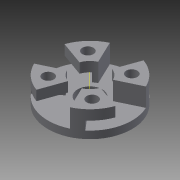
# Autodesk Inventor part: new male 4 bay con
Saved by Autodesk Inventor 2015 (Build 190159000, 159)
## iProperties
Created: 2014-11-16
Part Number: new male 4 bay con
Material: Generic
Document SubType Name: Modeling
Designer: ericd_000
Density: 1 g/cm^3
Appearance: Default
Author: ericd_000
Autodesk Inventor part; units mm, degrees
ref_plane "YZ Plane" through (0, 0, 0) normal (1, 0, 0) x (0, 1, 0)
ref_plane "XZ Plane" through (0, 0, 0) normal (0, 1, 0) x (-1, 0, 0)
ref_plane "XY Plane" through (0, 0, 0) normal (0, 0, 1) x (1, 0, 0)
sketch "Sketch1" plane through (0, 0, 0) normal (0, 0, 1) x (1, 0, 0)
  circle A0 centre (0, 0) radius 34
  dimension "d0" = 68
  constraints: 1 centre point, 1 coincident
  measures "d0" diameter of A0
extrude "Extrusion1" add sketch "Sketch1" along normal blind 6
sketch "Sketch2" plane through (0, 0, 6) normal (0, 0, 1) x (1, 0, 0)
  circle A0 centre (0, 0) radius 34
  circle A1 centre (0, 0) radius 34 projected
  line L0 (0, 0) -> (30.6997, 14.6126) construction
  line L1 (0, 0) -> (25.8716, 22.0604) construction
  line L2 (25.8716, 22.0604) -> (10.653, 9.0837)
  line L3 (30.6997, 14.6126) -> (12.641, 6.017)
  arc A2 (30.6997, 14.6126) -> (25.8716, 22.0604) centre (0, 0) ccw
  arc A3 (12.641, 6.017) -> (10.653, 9.0837) centre (0, 0) ccw
  dimension "d3" = 15
  dimension "d4" = 20
  constraints: 8 end point, 8 point on circle, 3 centre point, 3 concentric, 2 point on line, 1 coincident
  measures "d3" angle of L0 L1
  measures "d4" distance of L1.end L2.end
extrude "Extrusion2" add sketch "Sketch2" along normal blind 15 contours L3 A3 L2 A0 picked at (22.8031, 15.025)
sketch "Sketch3" plane through (10.653, 9.0837, 21) normal (-0.6488347, 0.7609293, 0) x (0.7609293, 0.6488347, 0)
  line L0 (0, 15) -> (0, 0) projected
  line L1 (20, 0) -> (0, 0)
  line L2 (0, 0) -> (0, 8)
  line L3 (0, 8) -> (20, 8)
  line L4 (20, 8) -> (20, 0)
  line L5 (-14, 25.2) -> (-14, -4.2) projected
  line L6 (-48, 15) -> (20, 15) projected
  point P0 (-14, 21)
  point P1 (18.8415, 15)
  dimension "d7" = 8
  dimension "d26" = 7
  constraints: 8 end point, 2 parallel, 1 horizontal, 1 perpendicular, 1 point on line
  measures "d7" distance between parallel lines of L3 L1
  measures "d26" distance between parallel lines of L6 L3
revolve "Revolution1" add sketch "Sketch3" angle 30 about axis through (0, 0, 6) along (0, 0, 1)
sketch "Sketch4" plane through (0, 0, 21) normal (0, 0, 1) x (1, 0, 0)
  circle A0 centre (16.0735, 17.8225) radius 4.5
  arc A1 (12.641, 6.017) -> (4.6839, 13.1932) centre (0, 0) ccw projected
  arc A2 (30.6997, 14.6126) -> (11.3753, 32.0406) centre (0, 0) ccw projected
  line L0 (12.641, 6.017) -> (30.6997, 14.6126) projected
  line L1 (4.6839, 13.1932) -> (11.3753, 32.0406) projected
  arc A3 (21.6704, 10.3148) -> (8.0296, 22.6169) centre (0, 0) ccw construction
  circle A4 centre (0, 0) radius 34 construction
  line L2 (22.7708, 25.2486) -> (18.7388, 20.7779) construction
  dimension "d12" = 9
  constraints: 5 point on circle, 2 centre point, 2 end point, 2 midpoint, 1 concentric, 1 line through centre, 1 point on line
  measures "d12" diameter of A0
extrude "Extrusion3" cut sketch "Sketch4" against normal blind 10 contours A0
pattern_circular "Circular Pattern2" count 4 over 360 about axis through (0, 0, 6) along (0, 0, 1) of "Revolution1", "Extrusion3", "Extrusion2"
sketch "Sketch5" plane through (0, 0, 0) normal (0, 0, -1) x (-1, 0, 0)
  circle A0 centre (0, 0) radius 10
  dimension "d23" = 20
  constraints: 1 centre point, 1 coincident
  measures "d23" diameter of A0
extrude "Extrusion4" cut sketch "Sketch5" against normal blind 10
body "Solid1"
